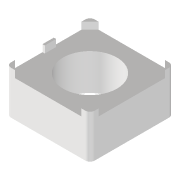
# Autodesk Inventor part: 00_VCM_M12
Saved by Autodesk Inventor 2022 (Build 260153000, 153)
## iProperties
Created: 2023-01-02
Part Number: 00_VCM_M12
Material: Generisch
Document SubType Name: Modeling
Designer: diederichbenedict
Density: 1 g/cm^3
Appearance: Vorgabe
Author: diederichbenedict
Autodesk Inventor part; units mm, degrees
ref_plane "YZ Plane" through (0, 0, 0) normal (1, 0, 0) x (0, 1, 0)
ref_plane "XZ Plane" through (0, 0, 0) normal (0, 1, 0) x (-1, 0, 0)
ref_plane "XY Plane" through (0, 0, 0) normal (0, 0, 1) x (1, 0, 0)
sketch "Skizze1" plane through (0, 0, 0) normal (0, 1, 0) x (-1, 0, 0)
  line L0 (-9, -9) -> (9, -9)
  line L1 (9, -9) -> (9, 9)
  line L2 (9, 9) -> (-9, 9)
  line L3 (-9, 9) -> (-9, -9)
  line L4 (-9, -9) -> (9, 9) construction
  line L5 (9, -9) -> (-9, 9) construction
  circle A0 centre (0, 0) radius 5.8
  dimension "d0" = 18
  dimension "d1" = 18
  dimension "d2" = 11.6
  constraints: 12 end point, 2 midpoint, 2 parallel, 1 centre point, 1 coincident, 1 horizontal, 1 perpendicular
  measures "d0" distance of L2.end L1.end
  measures "d1" distance of L1.end L0.end
  measures "d2" diameter of A0
extrude "Extrusion1" add sketch "Skizze1" along normal blind 7.8
sketch "Skizze2" plane through (0, 7.8, 0) normal (0, 1, 0) x (1, 0, 0)
  line L0 (-9, 9) -> (-9, -9) projected
  line L1 (-9, -9) -> (9, -9) projected
  line L2 (9, -9) -> (9, 9) projected
  line L3 (9, 9) -> (-9, 9) projected
  circle A0 centre (0, 0) radius 5.8 projected
  line L4 (-9, 9) -> (-9, -9) projected
  line L5 (-9, -7.1615) -> (-7.1615, -9)
  line L6 (-9, -7.1615) -> (-6.4, -7.1615) construction
  dimension "d5" = 45
  dimension "d6" = 1.3
  constraints: 4 end point, 2 point on line, 1 equal length, 1 horizontal
  measures "d5" angle of L5 L6
  measures "d6" distance from line of L5 L0.end
extrude "Extrusion2" add sketch "Skizze2" along normal blind 1.5 contours L5 L1 L0
pattern_circular "Runde Anordnung1" count 4 over 360 about axis through (0, 0, 0) along (0, 1, 0) of "Extrusion2"
fillet "Rundung1" radius 1 4 edges at (-9, 4.65, 9) (9, 4.65, 9) (9, 4.65, -9) (-9, 4.65, -9)
sketch "Skizze3" plane through (-9, 7.8, 7.1615) normal (-1, 0, 0) x (0, 0, 1)
  line L0 (-15.1615, -7.8) -> (-15.1615, 1.5) projected
  line L1 (-15.1615, -7.8) -> (0.8385, -7.8) projected
  line L2 (0.8385, 1.5) -> (0.8385, -7.8) projected
  line L3 (0, 1.5) -> (0.8385, 1.5) projected
  line L4 (0, 0) -> (0, 1.5) projected
  line L5 (-14.323, 0) -> (0, 0) projected
  line L6 (-14.323, 0) -> (-14.323, 1.5) projected
  line L7 (-15.1615, 1.5) -> (-14.323, 1.5) projected
  line L8 (-8.3736, -1.5) -> (-5.9495, -1.5)
  line L9 (-5.9495, -1.5) -> (-5.9495, 1.5)
  line L10 (-5.9495, 1.5) -> (-8.3736, 1.5)
  line L11 (-8.3736, 1.5) -> (-8.3736, -1.5)
  line L12 (-14.323, 0) -> (0, 0) projected
  line L13 (-8.3736, -1.5) -> (-5.9495, 1.5) construction
  line L14 (-5.9495, -1.5) -> (-8.3736, 1.5) construction
  point P0 (-7.1615, -7.8)
  point P1 (-7.1615, 0)
  constraints: 12 end point, 3 midpoint, 2 parallel, 1 horizontal, 1 perpendicular
extrude "Extrusion3" add sketch "Skizze3" against normal blind 0.5 contours L11 L10 L9 L5 | L5 L9 L8 L11
